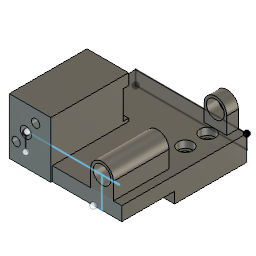
ソレノイド抑え (Autodesk Fusion 360 design; units mm, degrees)
Autodesk Fusion 360 part; units mm, degrees
note: some values were not read from the file. Set by a fixed rule: which sketch regions a step uses.
sketch "スケッチ1" plane through (0, 0, 0) normal (0, 0, 1) x (1, 0, 0)
  line L0 (0, 0) -> (40, 0)
  line L1 (40, 0) -> (40, 45)
  line L2 (40, 45) -> (0, 45)
  line L3 (0, 45) -> (0, 0)
  dimension "d1" = 40
  dimension "d2" = 45
  constraint horizontal L0
  constraint vertical L1
  constraint horizontal L2
  constraint vertical L3
  constraint coincident L0.start L3.end
  measures "d1" distance of L0.start L0.end
  measures "d2" distance of L0.start L2.end
extrude "押し出し1" add sketch "スケッチ1" along normal blind 5
sketch "スケッチ2" plane through (0, 0, 5) normal (0, 0, 1) x (-1, 0, 0)
  line L0 (0, -45) -> (0, 0)
  line L1 (0, 0) -> (-40, 0)
  line L2 (-40, 0) -> (-40, -45)
  line L3 (-40, -45) -> (0, -45)
  line L4 (0, 0) -> (-15, 0)
  line L5 (-15, 0) -> (-15, -27.5)
  line L6 (-15, -27.5) -> (0, -27.5)
  line L7 (0, -27.5) -> (0, 0)
  dimension "d5" = 15
  dimension "d6" = 27.5
  constraint horizontal L4
  constraint vertical L5
  constraint horizontal L6
  constraint vertical L7
  constraint coincident L0.end L1.start
  measures "d5" distance of L0.end L4.end
  measures "d6" distance of L0.end L6.end
extrude "押し出し2" add sketch "スケッチ2" along normal blind 15.2 contours L0 L1 L4 L5 L6 L7
sketch "スケッチ3" plane through (0, 0, 0) normal (-1, 0, 0) x (0, -1, 0)
  line L0 (-45, 0) -> (0, 0)
  line L1 (0, 0) -> (0, 20.2)
  line L2 (0, 20.2) -> (-27.5, 20.2)
  line L3 (-27.5, 20.2) -> (-27.5, 5)
  line L4 (-27.5, 5) -> (-45, 5)
  line L5 (-45, 5) -> (-45, 0)
  line L6 (0, 0) -> (-4, 0)
  line L7 (-4, 0) -> (-4, 20.2)
  line L8 (-4, 20.2) -> (0, 20.2)
  line L9 (0, 20.2) -> (0, 0)
  line L10 (-4, 5) -> (-24, 5)
  line L11 (-24, 5) -> (-24, 17.2)
  line L12 (-24, 17.2) -> (-4, 17.2)
  line L13 (-4, 17.2) -> (-4, 5)
  line L14 (-24, 5) -> (-25.5, 5)
  line L15 (-25.5, 5) -> (-25.5, 6)
  line L16 (-25.5, 6) -> (-24, 6)
  line L17 (-24, 6) -> (-24, 5)
  line L18 (-24, 17.2) -> (-25.5, 17.2)
  line L19 (-25.5, 17.2) -> (-25.5, 16.2)
  line L20 (-25.5, 16.2) -> (-24, 16.2)
  line L21 (-24, 16.2) -> (-24, 17.2)
  dimension "d9" = 4
  dimension "d10" = 20
  dimension "d11" = 12.2
  dimension "d12" = 1.5
  dimension "d13" = 1
  dimension "d14" = 1.5
  dimension "d15" = 1
  constraint horizontal L6
  constraint vertical L7
  constraint horizontal L8
  constraint vertical L9
  constraint coincident L0.end L1.start
  constraint horizontal L10
  constraint vertical L11
  constraint horizontal L12
  constraint vertical L13
  constraint coincident L7 L10.start
  constraint horizontal L14
  constraint vertical L15
  constraint horizontal L16
  constraint vertical L17
  constraint horizontal L18
  constraint vertical L19
  constraint horizontal L20
  constraint vertical L21
  measures "d9" distance of L0.end L6.end
  measures "d10" distance of L10.start L10.end
  measures "d11" distance of L10.start L12.end
  measures "d12" distance of L10.end L14.end
  measures "d13" distance of L10.end L16.end
  measures "d14" distance of L11.end L18.end
  measures "d15" distance of L11.end L20.end
extrude "押し出し3" cut sketch "スケッチ3" against normal blind 12 contours L7 L10 L11 L12 L13 L17 L21 | L11 L14 L15 L16 L17 | L11 L18 L19 L20 L21
sketch "スケッチ4" plane through (0, 0, 0) normal (-1, 0, 0) x (0, -1, 0)
  line L0 (-25.5, 16.2) -> (-25.5, 17.2)
  line L1 (-25.5, 17.2) -> (-4, 17.2)
  line L2 (-4, 17.2) -> (-4, 5)
  line L3 (-4, 5) -> (-25.5, 5)
  line L4 (-25.5, 5) -> (-25.5, 6)
  line L5 (-25.5, 6) -> (-24, 6)
  line L6 (-24, 6) -> (-24, 16.2)
  line L7 (-24, 16.2) -> (-25.5, 16.2)
  line L8 (-45, 0) -> (0, 0)
  line L9 (0, 0) -> (0, 20.2)
  line L10 (0, 20.2) -> (-27.5, 20.2)
  line L11 (-27.5, 20.2) -> (-27.5, 5)
  line L12 (-27.5, 5) -> (-45, 5)
  line L13 (-45, 5) -> (-45, 0)
  line L14 (-27.5, 6) -> (-25.5, 6)
  line L15 (-25.5, 6) -> (-25.5, 16.2)
  line L16 (-25.5, 16.2) -> (-27.5, 16.2)
  line L17 (-27.5, 16.2) -> (-27.5, 6)
  constraint horizontal L14
  constraint vertical L15
  constraint horizontal L16
  constraint vertical L17
  constraint coincident L0.start L7.end
  constraint coincident L11 L14.start
extrude "押し出し4" cut sketch "スケッチ4" against normal blind 15 contours L11 L14 L15 L16 L17
sketch "スケッチ6" plane through (12, 0, 0) normal (-1, 0, 0) x (0, -1, 0)
  line L0 (-4, 17.2) -> (-25.5, 17.2)
  line L1 (-25.5, 17.2) -> (-25.5, 16.2)
  line L2 (-25.5, 16.2) -> (-24, 16.2)
  line L3 (-24, 16.2) -> (-24, 6)
  line L4 (-24, 6) -> (-25.5, 6)
  line L5 (-25.5, 6) -> (-25.5, 5)
  line L6 (-25.5, 5) -> (-4, 5)
  line L7 (-4, 5) -> (-4, 17.2)
  line L8 (-25.5, 17.2) -> (-25, 17.2)
  line L9 (-25, 17.2) -> (-25, 16.2)
  line L10 (-25, 16.2) -> (-25.5, 16.2)
  line L11 (-25.5, 16.2) -> (-25.5, 17.2)
  line L12 (-25.5, 5) -> (-25, 5)
  line L13 (-25, 5) -> (-25, 6)
  line L14 (-25, 6) -> (-25.5, 6)
  line L15 (-25.5, 6) -> (-25.5, 5)
  dimension "d23" = 0.5
  dimension "d24" = 0.5
  constraint horizontal L8
  constraint vertical L9
  constraint horizontal L10
  constraint vertical L11
  constraint coincident L0.end L1.start
  constraint horizontal L12
  constraint vertical L13
  constraint horizontal L14
  constraint vertical L15
  constraint coincident L5.end L6.start
  measures "d23" distance of L0.end L8.end
  measures "d24" distance of L5.end L12.end
extrude "押し出し6" add sketch "スケッチ6" along normal blind 12 contours L0 L1 L2 L8 L9 L10 L11 | L4 L5 L6 L12 L13 L14 L15
sketch "スケッチ7" plane through (0, 0, 0) normal (-1, 0, 0) x (0, -1, 0)
  line L0 (-25, 6) -> (-24, 6)
  line L1 (-24, 6) -> (-24, 16.2)
  line L2 (-24, 16.2) -> (-25, 16.2)
  line L3 (-25, 16.2) -> (-25, 17.2)
  line L4 (-25, 17.2) -> (-4, 17.2)
  line L5 (-4, 17.2) -> (-4, 5)
  line L6 (-4, 5) -> (-25, 5)
  line L7 (-25, 5) -> (-25, 6)
  line L8 (-25.5, 6) -> (-27.5, 6)
  line L9 (-27.5, 6) -> (-27.5, 5)
  line L10 (-27.5, 5) -> (-45, 5)
  line L11 (-45, 5) -> (-45, 0)
  line L12 (-45, 0) -> (0, 0)
  line L13 (0, 0) -> (0, 20.2)
  line L14 (0, 20.2) -> (-27.5, 20.2)
  line L15 (-27.5, 20.2) -> (-27.5, 16.2)
  line L16 (-27.5, 16.2) -> (-25.5, 16.2)
  line L17 (-25.5, 16.2) -> (-25.5, 6)
  line L18 (-4, 5) -> (-3.5, 5)
  line L19 (-3.5, 5) -> (-3.5, 17.2)
  line L20 (-3.5, 17.2) -> (-4, 17.2)
  line L21 (-4, 17.2) -> (-4, 5)
  dimension "d27" = 0.5
  constraint horizontal L18
  constraint vertical L19
  constraint horizontal L20
  constraint vertical L21
  constraint coincident L5.end L6.start
  measures "d27" distance of L5.end L18.end
extrude "押し出し7" cut sketch "スケッチ7" against normal blind 12 contours L5 L18 L19 L20 L21
sketch "スケッチ8" plane through (0, 0, 0) normal (0, -1, 0) x (1, 0, 0)
  line L0 (0, 0) -> (40, 0)
  line L1 (40, 0) -> (40, 5)
  line L2 (40, 5) -> (15, 5)
  line L3 (15, 5) -> (15, 20.2)
  line L4 (15, 20.2) -> (0, 20.2)
  line L5 (0, 20.2) -> (0, 0)
  line L6 (0, 0) -> (15, 0)
  line L7 (15, 0) -> (15, 20.2)
  line L8 (15, 20.2) -> (0, 20.2)
  line L9 (0, 20.2) -> (0, 0)
  constraint horizontal L6
  constraint vertical L7
  constraint horizontal L8
  constraint vertical L9
  constraint coincident L3.end L4.start
  constraint coincident L0.start L5.end
extrude "押し出し8" add sketch "スケッチ8" along normal blind 0.5 contours L0 L3 L4 L5 L6 L7 L8 L9
sketch "スケッチ9" plane through (0, 25.5, 0) normal (0, 1, 0) x (-1, 0, 0)
  line L0 (0, 6) -> (0, 16.2)
  line L1 (0, 16.2) -> (-15, 16.2)
  line L2 (-15, 16.2) -> (-15, 6)
  line L3 (-15, 6) -> (0, 6)
  line L4 (-15, 16.2) -> (-12, 16.2)
  line L5 (-12, 16.2) -> (-12, 6)
  line L6 (-12, 6) -> (-15, 6)
  line L7 (-15, 6) -> (-15, 16.2)
  line L8 (0, 16.2) -> (-12, 6)
  line L9 (0, 6) -> (-12, 16.2)
  circle A0 centre (-6, 11.1) radius 2.5
  dimension "d32" = 5
  constraint horizontal L4
  constraint vertical L5
  constraint horizontal L6
  constraint vertical L7
  constraint coincident L3 L5.end
  constraint coincident L1.end L2.start
  constraint coincident L0.end L1.start
  constraint coincident L0.start L3.end
  constraint midpoint L9 A0.centre
  measures "d32" diameter of A0
extrude "押し出し9" cut sketch "スケッチ9" against normal blind 1.5 contours L8 L9 A0 | L8 L9 A0 | L8 L9 A0 | L8 L9 A0
sketch "スケッチ10" plane through (0, -0.5, 0) normal (0, -1, 0) x (1, 0, 0)
  line L0 (0, 20.2) -> (0, 0)
  line L1 (0, 0) -> (15, 0)
  line L2 (15, 0) -> (15, 20.2)
  line L3 (15, 20.2) -> (0, 20.2)
  line L4 (15, 20.2) -> (12, 20.2)
  line L5 (12, 20.2) -> (12, 0)
  line L6 (12, 0) -> (15, 0)
  line L7 (15, 0) -> (15, 20.2)
  line L8 (12, 5) -> (0, 5)
  line L9 (12, 20.2) -> (12, 17.2)
  line L10 (12, 17.2) -> (0, 17.2)
  line L11 (0, 5) -> (12, 17.2)
  line L12 (12, 5) -> (0, 17.2)
  circle A0 centre (6, 11.1) radius 2
  line L13 (0, 5) -> (2.5, 5)
  line L14 (2.5, 5) -> (2.5, 6.5)
  line L15 (2.5, 6.5) -> (0, 6.5)
  line L16 (0, 6.5) -> (0, 5)
  line L17 (12, 17.2) -> (9.5, 17.2)
  line L18 (9.5, 17.2) -> (9.5, 15.7)
  line L19 (9.5, 15.7) -> (12, 15.7)
  line L20 (12, 15.7) -> (12, 17.2)
  circle A1 centre (2.5, 6.5) radius 1.5
  circle A2 centre (9.5, 15.7) radius 1.5
  dimension "d35" = 3
  dimension "d36" = 4
  dimension "d37" = 2.5
  dimension "d38" = 1.5
  dimension "d39" = 2.5
  dimension "d40" = 1.5
  dimension "d41" = 3
  dimension "d42" = 3
  constraint horizontal L4
  constraint vertical L5
  constraint horizontal L6
  constraint vertical L7
  constraint coincident L1 L5.end
  constraint coincident L2.end L3.start
  constraint coincident L5 L8.start
  constraint coincident L0 L8.end
  constraint perpendicular L0 L8
  constraint coincident L5 L9.end
  constraint coincident L0 L10.end
  constraint perpendicular L0 L10
  constraint midpoint L11 A0.centre
  constraint horizontal L13
  constraint vertical L14
  constraint horizontal L15
  constraint vertical L16
  constraint horizontal L17
  constraint vertical L18
  constraint horizontal L19
  constraint vertical L20
  constraint coincident L14.end L15.start
  constraint coincident L18.end L19.start
  measures "d35" distance of L2.end L4.end
  measures "d36" diameter of A0
  measures "d37" distance of L8.end L13.end
  measures "d38" distance of L8.end L15.end
  measures "d39" distance of L9.end L17.end
  measures "d40" distance of L9.end L19.end
  measures "d41" diameter of A1
  measures "d42" diameter of A2
extrude "押し出し10" cut sketch "スケッチ10" against normal blind 4 contours L11 L18 L19 A2 | L11 L18 L19 A2 | L11 L12 A0 | L11 L12 A0 | L11 L15 A1 | L11 L15 A1 | L11 L19 A2 | L11 L19 A2 | L11 L12 A0 | L11 L12 A0 | L11 L14 L15 A1 | L11 L14 L15 A1
sketch "スケッチ11" plane through (0, 0, 0) normal (0, 0, -1) x (1, 0, 0)
  line L0 (0, 0.5) -> (0, -45)
  line L1 (0, -45) -> (40, -45)
  line L2 (40, -45) -> (40, 0)
  line L3 (40, 0) -> (15, 0)
  line L4 (15, 0) -> (15, 0.5)
  line L5 (15, 0.5) -> (0, 0.5)
  line L6 (40, -45) -> (36, -45)
  line L7 (36, -45) -> (36, -19)
  line L8 (36, -19) -> (40, -19)
  line L9 (40, -19) -> (40, -45)
  line L10 (36, -45) -> (29.8, -45)
  line L11 (29.8, -45) -> (25.8, -45)
  line L12 (25.8, -45) -> (25.8, -19)
  line L13 (25.8, -19) -> (29.8, -19)
  line L14 (29.8, -19) -> (29.8, -45)
  dimension "d45" = 4
  dimension "d46" = 26
  dimension "d47" = 6.2
  dimension "d48" = 4
  dimension "d49" = 26
  constraint horizontal L6
  constraint vertical L7
  constraint horizontal L8
  constraint vertical L9
  constraint coincident L1.end L2.start
  constraint perpendicular L7 L10
  constraint horizontal L11
  constraint vertical L12
  constraint horizontal L13
  constraint vertical L14
  measures "d45" distance of L1.end L6.end
  measures "d46" distance of L1.end L8.end
  measures "d47" distance of L6.end L10.end
  measures "d48" distance of L10.end L11.end
  measures "d49" distance of L10.end L13.end
extrude "押し出し11" add sketch "スケッチ11" along normal blind 4 contours L1 L11 L12 L13 L14 | L1 L2 L6 L7 L8 L9
sketch "スケッチ12" plane through (0, 0, 0) normal (0, 0, -1) x (1, 0, 0)
  line L0 (25.8, -45) -> (25.8, -19)
  line L1 (25.8, -19) -> (29.8, -19)
  line L2 (29.8, -19) -> (29.8, -45)
  line L3 (29.8, -45) -> (36, -45)
  line L4 (36, -45) -> (36, -19)
  line L5 (36, -19) -> (40, -19)
  line L6 (40, -19) -> (40, 0)
  line L7 (40, 0) -> (15, 0)
  line L8 (15, 0) -> (15, 0.5)
  line L9 (15, 0.5) -> (0, 0.5)
  line L10 (0, 0.5) -> (0, -45)
  line L11 (0, -45) -> (25.8, -45)
  line L12 (36, -45) -> (32.9, -45)
  line L13 (32.9, -45) -> (32.9, -19)
  line L14 (32.9, -19) -> (36, -19)
  line L15 (36, -19) -> (36, -45)
  line L16 (32.9, -45) -> (32.9, -37)
  line L17 (32.9, -37) -> (32.9, -29)
  circle A0 centre (32.9, -37) radius 1.65
  circle A1 centre (32.9, -29) radius 1.65
  dimension "d52" = 3.1
  dimension "d53" = 26
  dimension "d54" = 8
  dimension "d55" = 8
  dimension "d56" = 3.3
  dimension "d57" = 3.3
  constraint horizontal L12
  constraint vertical L13
  constraint horizontal L14
  constraint vertical L15
  constraint coincident L3.end L4.start
  constraint perpendicular L3 L16
  constraint parallel L13 L17
  constraint coincident L16.end L17.start
  constraint coincident L17.end A1.centre
  measures "d52" distance of L3.end L12.end
  measures "d53" distance of L3.end L4.end
  measures "d54" distance of L12.end L16.end
  measures "d55" distance of L16.end L17.end
  measures "d56" diameter of A0
  measures "d57" diameter of A1
extrude "押し出し12" cut sketch "スケッチ12" against normal blind 5 contours L13 L16 L17 A0 | L13 L16 L17 A0 | L13 L17 A1 | L13 L17 A1
sketch "スケッチ13" plane through (0, 0, 5) normal (0, 0, 1) x (-1, 0, 0)
  circle A0 centre (-32.9, -37) radius 1.65
  circle A1 centre (-32.9, -29) radius 1.65
  line L0 (-15, -27.5) -> (-15, 0)
  line L1 (-15, 0) -> (-40, 0)
  line L2 (-40, 0) -> (-40, -45)
  line L3 (-40, -45) -> (0, -45)
  line L4 (0, -45) -> (0, -27.5)
  line L5 (0, -27.5) -> (-15, -27.5)
  circle A2 centre (-32.9, -37) radius 2.75
  circle A3 centre (-32.9, -29) radius 2.75
  dimension "d60" = 5.5
  dimension "d61" = 5.5
  constraint concentric A0 A2
  constraint concentric A1 A3
  measures "d60" diameter of A2
  measures "d61" diameter of A3
extrude "押し出し13" cut sketch "スケッチ13" against normal blind 2.6 contours A2 | A3
sketch "スケッチ14" plane through (0, 45, 0) normal (0, 1, 0) x (-1, 0, 0)
  line L0 (-36, 0) -> (-29.8, 0)
  line L1 (-29.8, 0) -> (-29.8, -4)
  line L2 (-29.8, -4) -> (-25.8, -4)
  line L3 (-25.8, -4) -> (-25.8, 0)
  line L4 (-25.8, 0) -> (0, 0)
  line L5 (0, 0) -> (0, 5)
  line L6 (0, 5) -> (-40, 5)
  line L7 (-40, 5) -> (-40, -4)
  line L8 (-40, -4) -> (-36, -4)
  line L9 (-36, -4) -> (-36, 0)
  line L10 (-29.8, 0) -> (-32.9, 0)
  line L11 (-40, 5) -> (-40, 3.5)
  line L12 (-40, 3.5) -> (0, 3.5)
  line L13 (-32.9, 3.5) -> (-32.9, 8.05)
  circle A0 centre (-32.9, 8.05) radius 4.55
  dimension "d64" = 3.1
  dimension "d65" = 1.5
  dimension "d66" = 4.55
  dimension "d67" = 9.1
  constraint coincident L0.end L1.start
  constraint perpendicular L9 L10
  constraint coincident L6.end L7.start
  constraint perpendicular L6 L11
  constraint coincident L5 L12.end
  constraint perpendicular L5 L12
  constraint coincident L12 L13.start
  constraint perpendicular L6 L13
  constraint coincident L13.end A0.centre
  measures "d64" distance of L0.end L10.end
  measures "d65" distance of L6.end L11.end
  measures "d66" distance of L13.start L13.end
  measures "d67" diameter of A0
sketch "スケッチ16" plane through (0, 0, 0) normal (0, -1, 0) x (1, 0, 0)
  line L0 (15, 5) -> (15, 0)
  line L1 (15, 0) -> (40, 0)
  line L2 (40, 0) -> (40, 5)
  line L3 (40, 5) -> (15, 5)
extrude "押し出し16" add sketch "スケッチ16" against normal blind 20
sketch "スケッチ18" plane through (0, 0, 0) normal (0, -1, 0) x (1, 0, 0)
  line L0 (40, 5) -> (15, 5)
  line L1 (15, 5) -> (15, 0)
  line L2 (15, 0) -> (40, 0)
  line L3 (40, 0) -> (40, 5)
  circle A0 centre (32.9, 8.05) radius 3.12
  dimension "d82" = 6.24
  measures "d82" diameter of A0
sketch "スケッチ20" plane through (0, 0, 0) normal (-1, 0, 0) x (0, -1, 0)
  line L0 (-25.5, 6) -> (-27.5, 6)
  line L1 (-27.5, 6) -> (-27.5, 5)
  line L2 (-27.5, 5) -> (-45, 5)
  line L3 (-45, 5) -> (-45, 0)
  line L4 (-45, 0) -> (0.5, 0)
  line L5 (0.5, 0) -> (0.5, 20.2)
  line L6 (0.5, 20.2) -> (-27.5, 20.2)
  line L7 (-27.5, 20.2) -> (-27.5, 16.2)
  line L8 (-27.5, 16.2) -> (-25.5, 16.2)
  line L9 (-25.5, 16.2) -> (-25.5, 6)
  line L10 (-25, 17.2) -> (-3.5, 17.2)
  line L11 (-3.5, 17.2) -> (-3.5, 5)
  line L12 (-3.5, 5) -> (-25, 5)
  line L13 (-25, 5) -> (-25, 6)
  line L14 (-25, 6) -> (-24, 6)
  line L15 (-24, 6) -> (-24, 16.2)
  line L16 (-24, 16.2) -> (-25, 16.2)
  line L17 (-25, 16.2) -> (-25, 17.2)
  line L18 (-24, 6) -> (-25.5, 16.2)
  line L19 (-25.5, 6) -> (-24, 16.2)
  line L20 (-24.75, 11.1) -> (-24, 11.1)
  line L21 (-24, 11.1) -> (-24, 13.6)
  line L22 (-24, 13.6) -> (-24.75, 13.6)
  line L23 (-24.75, 13.6) -> (-24.75, 11.1)
  line L24 (-24, 13.6) -> (-25.5, 13.6)
  line L25 (-25.5, 13.6) -> (-25.5, 8.6)
  line L26 (-25.5, 8.6) -> (-24, 8.6)
  line L27 (-24, 8.6) -> (-24, 13.6)
  dimension "d88" = 2.5
  dimension "d89" = 5
  constraint coincident L14.end L15.start
  constraint coincident L8.end L9.start
  constraint coincident L0.start L9.end
  constraint coincident L15.end L16.start
  constraint horizontal L20
  constraint vertical L21
  constraint horizontal L22
  constraint vertical L23
  constraint coincident L15 L21.end
  constraint midpoint L18 L20.start
  constraint horizontal L24
  constraint vertical L25
  constraint horizontal L26
  constraint vertical L27
  measures "d88" distance of L20.start L22.end
  measures "d89" distance of L21.end L26.end
extrude "押し出し20" cut sketch "スケッチ20" against normal blind 6 contours L9 L18 L19 L24 L25 L26 | L18 L19 L26 | L15 L18 L20 L26 L27 | L19 L22 L23 L24 | L15 L19 L20 L21 L22 L24 L27 | L18 L23 L24
sketch "スケッチ21" plane through (0, 3.5, 0) normal (0, 1, 0) x (-1, 0, 0)
  line L0 (0, 5) -> (0, 17.2)
  line L1 (0, 17.2) -> (-9.5, 17.2)
  circle A0 centre (-9.5, 15.7) radius 1.5
  line L2 (-9.5, 17.2) -> (-12, 17.2)
  line L3 (-12, 17.2) -> (-12, 5)
  line L4 (-12, 5) -> (-2.5, 5)
  circle A1 centre (-2.5, 6.5) radius 1.5
  line L5 (-2.5, 5) -> (0, 5)
  circle A2 centre (-6, 11.1) radius 2
  line L6 (-6, 13.1) -> (0, 13.1)
  line L7 (-6, 9.1) -> (0, 9.1)
  constraint coincident A2 L6.start
  constraint coincident L0 L6.end
  constraint perpendicular L0 L6
  constraint coincident A2 L7.start
  constraint coincident L0 L7.end
  constraint perpendicular L0 L7
extrude "押し出し21" cut sketch "スケッチ21" against normal blind 1.5 contours L0 A2 L6 L7
sketch "スケッチ27" plane through (0, 45, 0) normal (0, 1, 0) x (-1, 0, 0)
  line L0 (-36, 0) -> (-29.8, 0)
  line L1 (-29.8, 0) -> (-29.8, -4)
  line L2 (-29.8, -4) -> (-25.8, -4)
  line L3 (-25.8, -4) -> (-25.8, 0)
  line L4 (-25.8, 0) -> (0, 0)
  line L5 (0, 0) -> (0, 5)
  line L6 (0, 5) -> (-40, 5)
  line L7 (-40, 5) -> (-40, -4)
  line L8 (-40, -4) -> (-36, -4)
  line L9 (-36, -4) -> (-36, 0)
  line L10 (-40, 5) -> (0, 5)
  line L11 (0, 5) -> (0, 0)
  line L12 (0, 0) -> (-40, 0)
  line L13 (-40, 0) -> (-40, 5)
  constraint horizontal L10
  constraint vertical L11
  constraint horizontal L12
  constraint vertical L13
  constraint coincident L4.end L5.start
  constraint coincident L6.end L7.start
move_face "面を移動1" to x (1, 0, 0) y (0, 1, 0) z (0, 0, 1) at (0, 1, 0) 6 faces at (34.5479, 37.0822, 1.6) (30.5269, 37.1366, 2.4) (30.1534, 37.1371, 3.2667) (34.5479, 29.0822, 1.6) (30.5269, 29.1366, 2.4) (30.1534, 29.1371, 3.2667)
sketch "スケッチ32" plane through (0, 0, 0) normal (0, -1, 0) x (1, 0, 0)
  line L0 (15, 5) -> (15, 0)
  line L1 (15, 0) -> (40, 0)
  line L2 (40, 0) -> (40, 5)
  line L3 (40, 5) -> (15, 5)
sketch "スケッチ33" plane through (0, -0.5, 0) normal (0, -1, 0) x (1, 0, 0)
  circle A0 centre (2.5, 6.5) radius 1.5
  circle A1 centre (6, 11.1) radius 2
  circle A2 centre (9.5, 15.7) radius 1.5
  line L0 (0, 20.2) -> (0, 0)
  line L1 (0, 0) -> (15, 0)
  line L2 (15, 0) -> (15, 20.2)
  line L3 (15, 20.2) -> (0, 20.2)
  line L4 (6, 11.1) -> (6, 5)
  constraint coincident A1.centre L4.start
  constraint vertical L4
sketch "スケッチ34" plane through (0, 0, 0) normal (0, -1, 0) x (1, 0, 0)
  line L0 (6, 11.1) -> (39, 11.1)
  line L1 (29.8, 0) -> (32.9, 0)
  line L2 (32.9, 0) -> (32.9, 11.1)
  line L3 (39, 11.1) -> (35.5, 11.1)
  dimension "d122" = 3.1
  constraint horizontal L0
  constraint horizontal L1
  constraint coincident L0 L2.end
  constraint perpendicular L0 L2
  constraint coincident L0 L3.end
  measures "d122" distance of L1.start L1.end
sketch "スケッチ35" plane through (0, 0, 0) normal (0, -1, 0) x (1, 0, 0)
  circle A0 centre (32.9, 11.1) radius 4.1
  line L0 (28.8, 11.1) -> (37, 11.1)
  line L1 (37, 11.1) -> (37, 5)
  line L2 (37, 5) -> (28.8, 5)
  line L3 (28.8, 5) -> (28.8, 11.1)
  dimension "d123" = 8.2
  constraint horizontal L0
  constraint vertical L1
  constraint horizontal L2
  constraint vertical L3
  constraint coincident A0 L0.start
  measures "d123" diameter of A0
extrude "押し出し29" add sketch "スケッチ35" against normal blind 20
sketch "スケッチ36" plane through (0, 0, 0) normal (0, -1, 0) x (1, 0, 0)
  line L0 (15, 5) -> (15, 0)
  line L1 (15, 0) -> (40, 0)
  line L2 (40, 0) -> (40, 5)
  line L3 (40, 5) -> (37, 5)
  line L4 (37, 5) -> (37, 11.1)
  arc A0 (37, 11.1) -> (28.8, 11.1) centre (32.9, 11.1) ccw
  line L5 (28.8, 11.1) -> (28.8, 5)
  line L6 (28.8, 5) -> (15, 5)
  circle A1 centre (32.9, 11.1) radius 3.2
  dimension "d126" = 6.4
  constraint concentric A0 A1
  measures "d126" diameter of A1
extrude "押し出し30" cut sketch "スケッチ36" against normal blind 20 contours A1
sketch "スケッチ37" plane through (0, 45, 0) normal (0, 1, 0) x (-1, 0, 0)
  circle A0 centre (-32.9, 11.1) radius 4.1
  line L0 (-37, 5) -> (-28.8, 5)
  line L1 (-28.8, 5) -> (-28.8, 11.1)
  line L2 (-28.8, 11.1) -> (-37, 11.1)
  line L3 (-37, 11.1) -> (-37, 5)
  dimension "d129" = 8.2
  constraint horizontal L0
  constraint vertical L1
  constraint horizontal L2
  constraint vertical L3
  constraint coincident A0 L1.end
  measures "d129" diameter of A0
extrude "押し出し31" add sketch "スケッチ37" against normal blind 4.2
sketch "スケッチ38" plane through (0, 45, 0) normal (0, 1, 0) x (-1, 0, 0)
  line L0 (-36, 0) -> (-29.8, 0)
  line L1 (-29.8, 0) -> (-29.8, -4)
  line L2 (-29.8, -4) -> (-25.8, -4)
  line L3 (-25.8, -4) -> (-25.8, 0)
  line L4 (-25.8, 0) -> (0, 0)
  line L5 (0, 0) -> (0, 5)
  line L6 (0, 5) -> (-28.8, 5)
  line L7 (-28.8, 5) -> (-28.8, 11.1)
  arc A0 (-28.8, 11.1) -> (-37, 11.1) centre (-32.9, 11.1) ccw
  line L8 (-37, 11.1) -> (-37, 5)
  line L9 (-37, 5) -> (-40, 5)
  line L10 (-40, 5) -> (-40, -4)
  line L11 (-40, -4) -> (-36, -4)
  line L12 (-36, -4) -> (-36, 0)
  circle A1 centre (-32.9, 11.1) radius 3.2
  dimension "d132" = 6.4
  constraint concentric A0 A1
  measures "d132" diameter of A1
extrude "押し出し32" cut sketch "スケッチ38" against normal blind 4.2 contours A1
